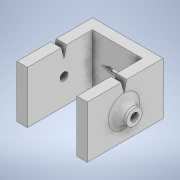
# Autodesk Inventor part: gaura_9mm_semn
Saved by Autodesk Inventor 2022.6 (Build 266554000, 554)
## iProperties
Created: 2026-01-08
Part Number: gaura_9mm_semn
Material: Generic
Document SubType Name: Modeling
Designer: Dragos Macovei
Density: 1 g/cm^3
Appearance: Default
Author: Dragos Macovei
Autodesk Inventor part; units mm, degrees
ref_plane "YZ Plane" through (0, 0, 0) normal (1, 0, 0) x (0, 1, 0)
ref_plane "XZ Plane" through (0, 0, 0) normal (0, 1, 0) x (-1, 0, 0)
ref_plane "XY Plane" through (0, 0, 0) normal (0, 0, 1) x (1, 0, 0)
sketch "Sketch1" plane through (0, 0, 0) normal (0, 1, 0) x (-1, 0, 0)
  line L0 (0, 0) -> (27, 0)
  line L1 (27, 0) -> (27, 29)
  line L2 (27, 29) -> (23, 29)
  line L3 (23, 29) -> (23, 4)
  line L4 (23, 4) -> (4, 4)
  line L5 (4, 4) -> (4, 29)
  line L6 (4, 29) -> (0, 29)
  line L7 (0, 29) -> (0, 0)
  point P0 (4, 16.5)
  point P1 (27, 14.5)
  point P2 (25, 29)
  dimension "d1" = 4
  dimension "d2" = 4
  dimension "d3" = 4
  dimension "d4" = 25
  dimension "d5" = 25
  dimension "d6" = 19
  constraints: 16 end point, 7 perpendicular, 3 midpoint, 1 horizontal
  measures "d1" distance from line of L7 point (4, 16.5)
  measures "d2" distance from line of point (27, 14.5) L3
  measures "d3" distance between parallel lines of L0 L4
  measures "d4" distance from line of L4 point (25, 29)
  measures "d5" distance from line of L4 L6.end
  measures "d6" distance between parallel lines of L5 L3
extrude "Extrusion1" add sketch "Sketch1" along normal blind 20
sketch "Sketch2" plane through (0, 0, 29) normal (1, 0, 0) x (0, 0, -1)
  point P0 (29, 0)
sketch "Sketch3" plane through (-4, 0, 4) normal (-1, 0, 0) x (0, 0, 1)
  line L0 (0, 0) -> (0, 20) projected
  line L1 (0, 10) -> (11, 10)
  circle A0 centre (11, 10) radius 1.5
  point P0 (-4, 0)
  dimension "d9" = 11
  dimension "d10" = 3
  constraints: 2 end point, 1 centre point, 1 coincident, 1 horizontal, 1 midpoint
  measures "d9" distance of L1.start L1.end
  measures "d10" diameter of A0
extrude "Extrusion2" cut sketch "Sketch3" along normal through all both and the other way through all
sketch "Sketch4" plane through (-27, 0, 0) normal (-1, 0, 0) x (0, 0, 1)
  circle A0 centre (15, 10) radius 1.5 projected
  line L0 (0, 0) -> (29, 0) projected
  line L1 (29, 0) -> (29, 20) projected
  line L2 (0, 20) -> (29, 20) projected
  line L3 (0, 0) -> (0, 20) projected
  circle A1 centre (15, 10) radius 1.5
  circle A2 centre (15, 10) radius 1.5 projected
  circle A3 centre (15, 10) radius 3
  point P0 (0, 0)
  dimension "d13" = 6
  constraints: 2 centre point, 2 coincident, 1 concentric
  measures "d13" diameter of A3
extrude "Extrusion3" add sketch "Sketch4" along normal blind 4 contours A3
fillet "Fillet1" radius 3 1 edges at (-27, 10, 12)
sketch "Sketch5" plane through (0, 0, 29) normal (1, 0, 0) x (0, 0, -1)
  circle A0 centre (14, 10) radius 3 projected
  circle A1 centre (14, 10) radius 1.5
  circle A2 centre (14, 10) radius 3
  point P0 (29, 0)
  dimension "d17" = 6
  constraints: 2 centre point, 2 coincident
  measures "d17" diameter of A2
extrude "Extrusion4" add sketch "Sketch5" along normal blind 4
fillet "Fillet2" radius 3 1 edges at (0, 10, 18)
sketch "Sketch6" plane through (0, 0, 29) normal (1, 0, 0) x (0, 0, -1)
  line L0 (0, 0) -> (29, 0) projected
  line L1 (29, 0) -> (29, 20) projected
  line L2 (0, 20) -> (29, 20) projected
  line L3 (0, 0) -> (0, 20) projected
  circle A0 centre (14, 10) radius 6 projected
  circle A1 centre (14, 10) radius 1.5 projected
  line L4 (14, 10) -> (14, 20)
  line L5 (14, 20) -> (15, 20)
  line L6 (0, 20) -> (29, 20) projected
  line L7 (14, 20) -> (13, 20)
  line L8 (13, 20) -> (14, 16)
  line L9 (15, 20) -> (14, 16)
  dimension "d21" = 1
  dimension "d22" = 1
  constraints: 10 end point, 4 point on line, 1 perpendicular, 1 vertical alignment, 1 other
  measures "d21" distance of L4.end L5.end
  measures "d22" distance of L4.end L7.end
extrude "Extrusion5" cut sketch "Sketch6" along normal through all both and the other way through all contours L2 L4 L8 | L9 L4 L2
sketch "Sketch7" plane through (0, 0, 0) normal (0, 0, -1) x (-1, 0, 0)
  line L0 (0, 0) -> (27, 0) projected
  line L1 (27, 0) -> (27, 20) projected
  line L2 (0, 20) -> (27, 20) projected
  line L3 (0, 0) -> (0, 20) projected
  line L4 (13.5, 10) -> (10.5, 10)
  line L5 (10.5, 10) -> (10.5, 9)
  line L6 (10.5, 9) -> (13.5, 9)
  line L7 (13.5, 9) -> (13.5, 10)
  line L8 (13.5, 10) -> (16.5, 10)
  line L9 (16.5, 10) -> (16.5, 9)
  line L10 (16.5, 9) -> (13.5, 9)
  line L11 (13.5, 9) -> (13.5, 10)
  line L12 (16.5, 10) -> (10.5, 10)
  line L13 (10.5, 10) -> (10.5, 11)
  line L14 (10.5, 11) -> (16.5, 11)
  line L15 (16.5, 11) -> (16.5, 10)
  dimension "d25" = 3
  dimension "d26" = 1
  dimension "d27" = 3
  dimension "d28" = 1
  dimension "d29" = 1
  constraints: 24 end point, 6 parallel, 3 horizontal, 3 perpendicular, 1 point on line
  measures "d25" distance of L6.end L5.end
  measures "d26" distance of L5.end L4.end
  measures "d27" distance of L9.end L10.end
  measures "d28" distance of L8.end L9.end
  measures "d29" distance of L12.end L13.end
extrude "Extrusion6" cut sketch "Sketch7" against normal through all contours L7 L6 L5 L4 | L8 L9 L10 L7 | L4 L13 L14 L15 L8
fillet "Fillet3" radius 3 7 edges at (-13.5, 11, 0) (-16.5, 9.5, 0) (-16.5, 10.5, 0) (-15, 9, 0) (-12, 9, 0) (-10.5, 9.5, 0) (-10.5, 10.5, 0) inverted yes
sketch "Sketch8" plane through (0, 0, 0) normal (0, 0, -1) x (-1, 0, 0)
  line L0 (16.5, 9) -> (16.5, 11) projected
  line L1 (10.5, 11) -> (10.5, 9) projected
  line L2 (7.5, 14) -> (7.5, 6) projected
  line L3 (19.5, 6) -> (19.5, 14) projected
  line L4 (16.5, 11) -> (19.5, 10)
  line L5 (16.5, 9) -> (19.5, 10)
  line L6 (16.5, 11) -> (10.5, 11) projected
  line L7 (10.5, 11) -> (7.5, 10)
  line L8 (7.5, 10) -> (10.5, 9)
  point P0 (0, 0)
  point P1 (16.5, 10)
  point P2 (10.5, 10)
  constraints: 8 end point, 4 midpoint, 2 parallel
extrude "Extrusion7" cut sketch "Sketch8" along normal through all both and the other way through all
body "Solid1"
